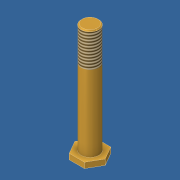
# Autodesk Inventor part: Bolzen
Saved by Autodesk Inventor 2016 (Build 200138000, 138)
## iProperties
Created: 2015-09-09
Part Number: Bolzen
Material: Messing, weicher Gelbton
Document SubType Name: Modeling
Designer: 4ndreas
Density: 8.47 g/cm^3
Appearance: Messing - satiniert
Mass: 23.4236 g
Surface Area: 16.3999 cm^2
Volume: 2.76548 cm^3
Author: 4ndreas
Autodesk Inventor part; units mm, degrees
ref_plane "YZ Plane" through (0, 0, 0) normal (1, 0, 0) x (0, 1, 0)
ref_plane "XZ Plane" through (0, 0, 0) normal (0, 1, 0) x (-1, 0, 0)
ref_plane "XY Plane" through (0, 0, 0) normal (0, 0, 1) x (1, 0, 0)
sketch "Skizze1" plane through (0, 0, 0) normal (0, 0, 1) x (1, 0, 0)
  circle A0 centre (0, 0) radius 6
  dimension "d0" = 12
  constraints: 1 centre point, 1 coincident
  measures "d0" diameter of A0
extrude "Extrusion1" add sketch "Skizze1" along normal blind 2.5
sketch "Skizze2" plane through (0, 0, 2.5) normal (0, 0, 1) x (1, 0, 0)
  circle A0 centre (0, 0) radius 4
  dimension "d3" = 8
  constraints: 1 centre point, 1 coincident
  measures "d3" diameter of A0
extrude "Extrusion2" add sketch "Skizze2" along normal blind 50
sketch "Skizze3" plane through (0, 0, 0) normal (0, 0, -1) x (-1, 0, 0)
  circle A0 centre (0, 0) radius 3
  dimension "d6" = 6
  constraints: 1 centre point, 1 coincident
  measures "d6" diameter of A0
extrude "Extrusion3" cut sketch "Skizze3" against normal blind 2
sketch "Skizze4" plane through (0, 0, 0) normal (0, 0, -1) x (-1, 0, 0)
  line L0 (3.4641, 6) -> (6.9282, 0)
  line L1 (6.9282, 0) -> (3.4641, -6)
  line L2 (3.4641, -6) -> (-3.4641, -6)
  line L3 (-3.4641, -6) -> (-6.9282, 0)
  line L4 (-6.9282, 0) -> (-3.4641, 6)
  line L5 (-3.4641, 6) -> (3.4641, 6)
  circle A0 centre (0, 0) radius 3 projected
  dimension "d9" = 12
  constraints: 12 end point, 1 coincident, 1 horizontal, 13 other
  measures "d9" distance between parallel lines of L2 L5
extrude "Extrusion4" add sketch "Skizze4" against normal up to surface (2.5 mm away)
chamfer "Fase1" distance 0.5 angle 45 1 edges at (-4, 0, 52.5)
thread "Gewinde1" size "M8x1.25" class "6g" standard "ANSI Metric M Profile" length 15
